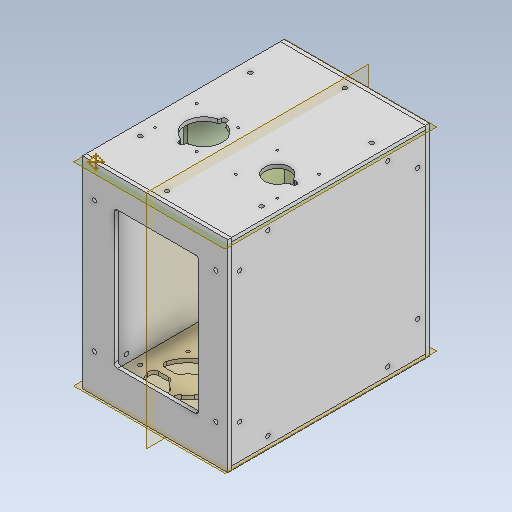
# Autodesk Inventor part: Front face
Saved by Autodesk Inventor 2020 (Build 240168000, 168)
## iProperties
Created: 2020-04-08
Part Number: Front face
Material: Generic
Document SubType Name: Modeling
Designer: angusaitken
Density: 1 g/cm^3
Appearance: Default
Author: angusaitken
Autodesk Inventor part; units mm, degrees
ref_plane "YZ Plane" through (0, 0, 0) normal (1, 0, 0) x (0, 1, 0)
ref_plane "XZ Plane" through (0, 0, 0) normal (0, 1, 0) x (-1, 0, 0)
sketch "Sketch1" plane through (0, 0, 0) normal (0, 0, 1) x (1, 0, 0)
  line L0 (0, 0) -> (170.5, 0)
  line L1 (170.5, 0) -> (170.5, 240.5)
  line L2 (170.5, 240.5) -> (0, 240.5)
  line L3 (0, 240.5) -> (0, 0)
  line L4 (175.25, 245.25) -> (175.25, -4.75)
  line L5 (175.25, -4.75) -> (-4.75, -4.75)
  line L6 (-4.75, -4.75) -> (-4.75, 245.25)
  line L7 (-4.75, 245.25) -> (175.25, 245.25)
  line L8 (137.1, 204.87) -> (137.1, 42.67) projected
  line L9 (137.1, 204.87) -> (137.1, 42.67) projected
  arc A0 (137.1, 204.87) -> (135.1, 206.87) centre (135.1, 204.87) ccw projected
  line L10 (38.5, 206.87) -> (135.1, 206.87) projected
  arc A1 (38.5, 206.87) -> (36.5, 204.87) centre (38.5, 204.87) ccw projected
  line L11 (36.5, 42.67) -> (36.5, 204.87) projected
  arc A2 (36.5, 42.67) -> (38.5, 40.67) centre (38.5, 42.67) ccw projected
  line L12 (135.1, 40.67) -> (38.5, 40.67) projected
  arc A3 (135.1, 40.67) -> (137.1, 42.67) centre (135.1, 42.67) ccw projected
  arc A4 (139.1, 204.87) -> (135.1, 208.87) centre (135.1, 204.87) ccw
  line L13 (135.1, 208.87) -> (38.5, 208.87)
  arc A5 (38.5, 208.87) -> (34.5, 204.87) centre (38.5, 204.87) ccw
  line L14 (34.5, 204.87) -> (34.5, 42.67)
  arc A6 (34.5, 42.67) -> (38.5, 38.67) centre (38.5, 42.67) ccw
  line L15 (38.5, 38.67) -> (135.1, 38.67)
  arc A7 (135.1, 38.67) -> (139.1, 42.67) centre (135.1, 42.67) ccw
  line L16 (139.1, 204.87) -> (139.1, 42.67)
  dimension "d0" = 170.5
  dimension "d1" = 240.5
  dimension "d2" = 4.75
  dimension "d5" = 2
  dimension "d6" = 2
  constraints: 24 end point, 8 point on circle, 5 parallel, 4 centre point, 2 perpendicular, 1 horizontal, 9 other
  measures "d0" distance of L2.end L1.end
  measures "d1" distance of L1.end L0.end
  measures "d2" distance between parallel lines of L1 L4
  measures "d5" distance between parallel lines of L10 L13
  measures "d6" distance between parallel lines of L8 L16
extrude "Extrusion1" add sketch "Sketch1" along normal blind 4.75 contours L3 L2 L1 L0 | L4 L5 L6 L7 | L8 A3 L12 A2 L11 A1 L10 A0 | L16 A7 L15 A6 L14 A5 L13 A4
sketch "Sketch2" plane through (0, 0, 0) normal (0, 0, -1) x (-1, 0, 0)
  line L0 (-137.1, 204.87) -> (-137.1, 42.67) projected
  line L1 (-137.1, 204.87) -> (-137.1, 42.67) projected
  line L2 (-137.1, 204.87) -> (-137.1, 42.67) projected
  arc A0 (-135.1, 206.87) -> (-137.1, 204.87) centre (-135.1, 204.87) ccw projected
  line L3 (-38.5, 206.87) -> (-135.1, 206.87) projected
  arc A1 (-36.5, 204.87) -> (-38.5, 206.87) centre (-38.5, 204.87) ccw projected
  line L4 (-36.5, 42.67) -> (-36.5, 204.87) projected
  arc A2 (-38.5, 40.67) -> (-36.5, 42.67) centre (-38.5, 42.67) ccw projected
  line L5 (-135.1, 40.67) -> (-38.5, 40.67) projected
  arc A3 (-137.1, 42.67) -> (-135.1, 40.67) centre (-135.1, 42.67) ccw projected
  line L6 (-139.1, 204.87) -> (-139.1, 42.67)
  arc A4 (-135.1, 208.87) -> (-139.1, 204.87) centre (-135.1, 204.87) ccw
  line L7 (-135.1, 208.87) -> (-38.5, 208.87)
  arc A5 (-34.5, 204.87) -> (-38.5, 208.87) centre (-38.5, 204.87) ccw
  line L8 (-34.5, 204.87) -> (-34.5, 42.67)
  arc A6 (-38.5, 38.67) -> (-34.5, 42.67) centre (-38.5, 42.67) ccw
  line L9 (-38.5, 38.67) -> (-135.1, 38.67)
  arc A7 (-139.1, 42.67) -> (-135.1, 38.67) centre (-135.1, 42.67) ccw
  point P0 (0, 0)
  point P1 (-139.1, 204.87)
  dimension "d9" = 2
  dimension "d10" = 2
  constraints: 8 end point, 8 point on circle, 4 centre point, 1 parallel, 6 other
  measures "d9" distance between parallel lines of L0 L6
  measures "d10" distance between parallel lines of L3 L7
extrude "Extrusion2" cut sketch "Sketch2" against normal through all contours A0 L3 A1 L4 A2 L5 A3 L0 | A4 L7 A5 L8 A6 L9 A7 L6
sketch "Sketch3" plane through (0, 0, 0) normal (0, 0, -1) x (-1, 0, 0)
  line L0 (-135.1, 208.87) -> (-38.5, 208.87) projected
  arc A0 (-34.5, 204.87) -> (-38.5, 208.87) centre (-38.5, 204.87) ccw projected
  line L1 (-34.5, 204.87) -> (-34.5, 42.67) projected
  arc A1 (-38.5, 38.67) -> (-34.5, 42.67) centre (-38.5, 42.67) ccw projected
  line L2 (-38.5, 38.67) -> (-135.1, 38.67) projected
  arc A2 (-139.1, 42.67) -> (-135.1, 38.67) centre (-135.1, 42.67) ccw projected
  line L3 (-139.1, 42.67) -> (-139.1, 204.87) projected
  arc A3 (-135.1, 208.87) -> (-139.1, 204.87) centre (-135.1, 204.87) ccw projected
  line L4 (4.75, -4.75) -> (-175.25, -4.75) projected
  line L5 (4.75, 245.25) -> (4.75, -4.75) projected
  line L6 (-175.25, 245.25) -> (4.75, 245.25) projected
  line L7 (-175.25, -4.75) -> (-175.25, 245.25) projected
  line L8 (-170.5, 240.5) -> (0, 240.5)
  line L9 (0, 240.5) -> (0, 0)
  line L10 (0, 0) -> (-170.5, 0)
  line L11 (-170.5, 0) -> (-170.5, 240.5)
  point P0 (0, 0)
  dimension "d11" = 4.75
  constraints: 8 end point, 3 other
  measures "d11" distance between parallel lines of L7 L11
ref_plane "Work Plane1" through (152.5168, 19.9337, -238.5381) normal (0, 0, -1) x (0, 1, 0)
extrude "Extrusion3" add sketch "Sketch3" along normal up to surface (238.5381 mm away) separate body contours L4 L7 L6 L5
ref_plane "Work Plane2" through (0, 240.5, 0) normal (0, -1, 0) x (1, 0, 0)
split body "Split1" result two bodies by plane through (0, 240.5, 0) normal (0, -1, 0) bodies 2 first body at (174.75, 158.75, -159.0254)
ref_plane "Work Plane3" through (0, 0, 0) normal (0, 1, 0) x (1, 0, 0)
split body "Split2" result two bodies by plane through (0, 0, 0) normal (0, 1, 0) bodies 3 first body at (174.75, 160.3333, -79.5127) (-0.5, 160.3333, -79.5127)
sketch "Sketch4" plane through (175.25, 240.5, -238.5381) normal (0, 0, -1) x (-1, 0, 0)
  line L0 (40.15, -31.63) -> (136.75, -31.63) projected
  arc A0 (140.75, -35.63) -> (136.75, -31.63) centre (136.75, -35.63) ccw projected
  line L1 (140.75, -35.63) -> (140.75, -197.83) projected
  arc A1 (136.75, -201.83) -> (140.75, -197.83) centre (136.75, -197.83) ccw projected
  line L2 (136.75, -201.83) -> (40.15, -201.83) projected
  arc A2 (36.15, -197.83) -> (40.15, -201.83) centre (40.15, -197.83) ccw projected
  line L3 (36.15, -197.83) -> (36.15, -35.63) projected
  arc A3 (40.15, -31.63) -> (36.15, -35.63) centre (40.15, -35.63) ccw projected
  line L4 (180, -245.25) -> (0, -245.25) projected
  line L5 (180, 4.75) -> (180, -245.25) projected
  line L6 (0, 4.75) -> (180, 4.75) projected
  line L7 (0, -245.25) -> (0, 4.75) projected
  point P0 (175.25, -240.5)
extrude "Extrusion4" add sketch "Sketch4" along normal blind 4.75 separate body contours L0 A0 L1 A1 L2 A2 L3 A3 | L4 L7 L6 L5
sketch "Sketch5" plane through (0, 0, 4.75) normal (0, 0, 1) x (1, 0, 0)
  line L0 (38.5, 208.87) -> (135.1, 208.87) projected
  arc A0 (139.1, 204.87) -> (135.1, 208.87) centre (135.1, 204.87) ccw projected
  line L1 (139.1, 204.87) -> (139.1, 42.67) projected
  arc A1 (135.1, 38.67) -> (139.1, 42.67) centre (135.1, 42.67) ccw projected
  line L2 (135.1, 38.67) -> (38.5, 38.67) projected
  arc A2 (34.5, 42.67) -> (38.5, 38.67) centre (38.5, 42.67) ccw projected
  line L3 (34.5, 42.67) -> (34.5, 204.87) projected
  arc A3 (38.5, 208.87) -> (34.5, 204.87) centre (38.5, 204.87) ccw projected
  line L4 (-4.75, -4.75) -> (175.25, -4.75) projected
  line L5 (175.25, -4.75) -> (175.25, 245.25) projected
  line L6 (175.25, 245.25) -> (-4.75, 245.25) projected
  line L7 (-4.75, 245.25) -> (-4.75, -4.75) projected
  line L8 (10, 10) -> (160.5, 10)
  line L9 (160.5, 10) -> (160.5, 230.5)
  line L10 (160.5, 230.5) -> (10, 230.5)
  line L11 (10, 230.5) -> (10, 10)
  circle A4 centre (10, 204.87) radius 2.6
  circle A5 centre (160.5, 204.87) radius 2.6
  circle A6 centre (10, 42.67) radius 2.6
  circle A7 centre (160.5, 42.67) radius 2.6
  point P0 (0, 0)
  dimension "d18" = 14.75
  dimension "d19" = 5.2
  dimension "d20" = 5.2
  dimension "d21" = 5.2
  dimension "d22" = 5.2
  constraints: 8 end point, 4 centre point, 4 point on line, 3 other
  measures "d18" distance between parallel lines of L7 L11
  measures "d19" diameter of A4
  measures "d20" diameter of A5
  measures "d21" diameter of A6
  measures "d22" diameter of A7
extrude "Extrusion5" cut sketch "Sketch5" against normal through all contours A6 L11 | L11 A6 | A7 L9 | L9 A7 | A4 L11 | L11 A4 | A5 L9 | L9 A5 bodies 1 7
sketch "Sketch6" plane through (-4.75, 240.5, -238.5381) normal (-1, 0, 0) x (0, 0, 1)
  line L0 (0, 0) -> (0, -240.5) projected
  line L1 (238.5381, -240.5) -> (0, -240.5) projected
  line L2 (238.5381, -240.5) -> (238.5381, 0) projected
  line L3 (0, 0) -> (238.5381, 0) projected
  line L4 (0, 0) -> (0, -240.5) projected
  line L5 (228.5381, -10) -> (228.5381, -230.5)
  line L6 (228.5381, -230.5) -> (10, -230.5)
  line L7 (10, -230.5) -> (10, -10)
  line L8 (10, -10) -> (228.5381, -10)
  line L9 (243.2881, -33.03) -> (243.2881, -38.23) projected
  line L10 (243.2881, -195.23) -> (243.2881, -200.43) projected
  circle A0 centre (228.5381, -35.63) radius 2.6
  circle A1 centre (228.5381, -197.83) radius 2.6
  circle A2 centre (10, -197.83) radius 2.6
  circle A3 centre (10, -35.63) radius 2.6
  circle A4 centre (45, -230.5) radius 2.6
  circle A5 centre (193.5381, -230.5) radius 2.6
  circle A6 centre (45, -10) radius 2.6
  circle A7 centre (193.5381, -10) radius 2.6
  point P0 (238.5381, -240.5)
  point P1 (119.269, -120.25)
  dimension "d25" = 10
  dimension "d26" = 5.2
  dimension "d27" = 5.2
  dimension "d28" = 5.2
  dimension "d29" = 5.2
  dimension "d30" = 5.2
  dimension "d31" = 5.2
  dimension "d32" = 35
  dimension "d33" = 35
  dimension "d34" = 5.2
  dimension "d35" = 5.2
  constraints: 8 centre point, 8 end point, 6 point on line, 3 other
  measures "d25" distance between parallel lines of L3 L8
  measures "d26" diameter of A0
  measures "d27" diameter of A1
  measures "d28" diameter of A2
  measures "d29" diameter of A3
  measures "d30" diameter of A4
  measures "d31" diameter of A5
  measures "d32" distance of L6.end A4.centre
  measures "d33" distance of L5.end A5.centre
  measures "d34" diameter of A6
  measures "d35" diameter of A7
extrude "Extrusion6" cut sketch "Sketch6" against normal through all contours A0 L5 | L5 A0 | A7 L8 | L8 A7 | A1 L5 | L5 A1 | A6 L8 | L8 A6 | A5 L6 | L6 A5 | A3 L7 | L7 A3 | A4 L6 | L6 A4 | A2 L7 | L7 A2 bodies 5
move or copy body "Move Body1" bodies to move or copy 7 copy no translate (0, 0, -1.947)
thicken "Thicken1" operation add thickness 1.947 both sides no extend neighbours yes toward (0, 0, -1) bodies 5 faces at (-1.5833, 160.3333, -238.5381)
move faces "Move1" translate (0, 0, -1.947) faces at (113.6667, 243.6667, -238.5381)
move faces "Move2" translate (0, 0, -1.947) faces at (56.8333, -3.1667, -238.5381)
move faces "Move3" translate (0, 0, -1.947) faces at (173.6667, 160.3333, -238.5381)
move faces "Move4" translate (0, 0, -1.947) faces at (172.0833, 40.1727, -229.2615)
move faces "Move5" translate (0, 0, -1.947) faces at (172.0833, 202.3727, -229.2615)
move faces "Move6" translate (0, 0, -1.947) faces at (-1.5833, 202.3727, -229.2615) (-1.5833, 40.1727, -229.2615)
sketch "Sketch7" plane through (-4.75, -4.75, 0) normal (0, -1, 0) x (1, 0, 0)
  circle A0 centre (14.7449, -9.98) radius 4.725
  circle A1 centre (165.2551, -9.98) radius 4.725
  circle A2 centre (165.2551, -230.4902) radius 2.6
  circle A3 centre (14.7449, -230.4902) radius 2.6
  point P0 (4.75, 0)
  constraints: 4 centre point, 8 other
hole "Hole1" at (160.5051, -4.75, -9.98) at (9.9949, -4.75, -9.98) at (9.9949, -4.75, -230.4902) at (160.5051, -4.75, -230.4902) direction (0, 1, 0) diameter 4.2 end through all bodies 6
ref_plane "Work Plane4" through (86.8, 42.67, 0) normal (1, 0, 0) x (0, 0, -1)
sketch "Sketch10" plane through (175.25, 245.25, -245.2351) normal (0, 0, -1) x (-1, 0, 0)
  circle A0 centre (85.2205, -159.8102) radius 42.45
  circle A1 centre (85.2205, -107.3602) radius 2.4
  circle A2 centre (39.7975, -186.0352) radius 2.4
  circle A3 centre (130.6435, -186.0352) radius 2.4
  point P0 (175.25, -245.25)
  constraints: 4 centre point, 8 other
extrude "Extrusion9" cut sketch "Sketch10" against normal through all bodies 7
sketch "Sketch11" plane through (-4.75, 0, 0) normal (-1, 0, 0) x (0, 0, 1)
  arc A0 (-158.1352, 97.3397) -> (-162.885, 92.5899) centre (-158.1352, 92.5899) ccw
  line L0 (-158.1352, 97.3397) -> (-143.835, 97.3397)
  arc A1 (-139.0852, 92.5899) -> (-143.835, 97.3397) centre (-143.835, 92.5899) ccw
  line L1 (-139.0852, 92.5899) -> (-139.0852, 78.2897)
  arc A2 (-143.835, 73.5399) -> (-139.0852, 78.2897) centre (-143.835, 78.2897) ccw
  line L2 (-143.835, 73.5399) -> (-158.1352, 73.5399)
  arc A3 (-162.885, 78.2897) -> (-158.1352, 73.5399) centre (-158.1352, 78.2897) ccw
  line L3 (-162.885, 78.2897) -> (-162.885, 92.5899)
  line L4 (-143.835, 97.8397) -> (-158.1352, 97.8397)
  arc A4 (-158.1352, 97.8397) -> (-163.385, 92.5899) centre (-158.1352, 92.5899) ccw
  line L5 (-163.385, 92.5899) -> (-163.385, 78.2897)
  arc A5 (-163.385, 78.2897) -> (-158.1352, 73.0399) centre (-158.1352, 78.2897) ccw
  line L6 (-158.1352, 73.0399) -> (-143.835, 73.0399)
  arc A6 (-143.835, 73.0399) -> (-138.5852, 78.2897) centre (-143.835, 78.2897) ccw
  line L7 (-138.5852, 78.2897) -> (-138.5852, 92.5899)
  arc A7 (-138.5852, 92.5899) -> (-143.835, 97.8397) centre (-143.835, 92.5899) ccw
  point P0 (0, 0)
  dimension "d79" = 0.5
  constraints: 16 end point, 16 point on circle, 8 centre point, 27 other
  measures "d79" distance between parallel lines of L0 L4
extrude "Extrusion10" cut sketch "Sketch11" against normal blind 10 contours L0 A1 L1 A2 L2 A3 L3 A0 | A7 L7 A6 L6 A5 L5 A4 L4 bodies 5
sketch "Sketch12" plane through (-4.75, 0, 0) normal (-1, 0, 0) x (0, 0, 1)
  line L0 (-120.9351, 195.1795) -> (-120.9351, 219.9795)
  line L1 (-120.9351, 219.9795) -> (-68.5351, 219.9795)
  line L2 (-68.5351, 219.9795) -> (-68.5351, 195.1795)
  line L3 (-68.5351, 195.1795) -> (-120.9351, 195.1795)
  point P0 (0, 0)
  constraints: 8 end point, 2 horizontal, 2 vertical, 4 other
extrude "Extrusion11" cut sketch "Sketch12" against normal blind 10 bodies 5
sketch "Sketch13" plane through (-4.75, 245.25, 0) normal (0, 1, 0) x (1, 0, 0)
  circle A0 centre (39.495, 94.7351) radius 12.65
  circle A1 centre (140.5, 94.7351) radius 12.65
  point P0 (4.75, 0)
  constraints: 2 centre point, 4 other
hole "Hole2" at (34.745, 245.25, -94.7351) at (135.75, 245.25, -94.7351) direction (0, -1, 0) diameter 31 end through all bodies 4
sketch "Sketch14" plane through (-4.75, 245.25, 0) normal (0, 1, 0) x (1, 0, 0)
  circle A0 centre (65.245, 68.9851) radius 1.6
  circle A1 centre (13.745, 68.9851) radius 1.6
  circle A2 centre (65.245, 120.4851) radius 1.6
  circle A3 centre (13.745, 120.4851) radius 1.6
  circle A4 centre (166.25, 120.4851) radius 1.6
  circle A5 centre (114.75, 120.4851) radius 1.6
  circle A6 centre (114.75, 68.9851) radius 1.6
  circle A7 centre (166.25, 68.9851) radius 1.6
  point P0 (4.75, 0)
  constraints: 8 centre point, 16 other
hole "Hole3" at (8.995, 245.25, -120.4851) at (60.495, 245.25, -120.4851) at (60.495, 245.25, -68.9851) at (8.995, 245.25, -68.9851) at (110, 245.25, -68.9851) at (161.5, 245.25, -68.9851) at (161.5, 245.25, -120.4851) at (110, 245.25, -120.4851) direction (0, -1, 0) diameter 2.8 end through all bodies 4
sketch "Sketch15" plane through (-4.75, 245.25, 0) normal (0, 1, 0) x (1, 0, 0)
  circle A0 centre (160.7871, 95.5911) radius 2.1
  line L0 (160.7871, 95.5911) -> (150.7871, 95.5911) construction
  line L1 (160.7871, 98.7156) -> (150.7871, 98.7156)
  line L2 (150.7871, 92.4666) -> (160.7871, 92.4666)
  arc A1 (160.7871, 92.4666) -> (160.7871, 98.7156) centre (160.7871, 95.5911) ccw
  arc A2 (150.7871, 98.7156) -> (150.7871, 92.4666) centre (150.7871, 95.5911) ccw
  point P0 (4.75, 0)
  point P1 (155.7871, 95.5911)
  dimension "d98" = 10
  constraints: 8 end point, 4 point on circle, 4 tangent, 3 centre point, 1 horizontal, 1 midpoint, 1 parallel, 2 other
  measures "d98" distance of L0.start L0.end
extrude "Extrusion12" cut sketch "Sketch15" against normal blind 10 contours A0 | A1 L2 A2 L1 bodies 4
fillet "Fillet1" radius 4 2 edges at (150.7302, 242.875, -98.7156) (151.0831, 242.875, -92.4666)
sketch "Sketch16" plane through (-4.75, -4.75, 0) normal (0, -1, 0) x (1, 0, 0)
  circle A0 centre (30.018, -96.0748) radius 2.5
  circle A1 centre (30.018, -24.5748) radius 2.5
  circle A2 centre (101.518, -24.5748) radius 2.5
  circle A3 centre (101.518, -96.0748) radius 2.5
  point P0 (4.75, 0)
  constraints: 4 centre point, 8 other
hole "Hole4" at (25.268, -4.75, -96.0748) at (25.268, -4.75, -24.5748) at (96.768, -4.75, -24.5748) at (96.768, -4.75, -96.0748) direction (0, 1, 0) diameter 4 depth 8 bodies 6
sketch "Sketch17" plane through (-4.75, -4.75, 0) normal (0, -1, 0) x (1, 0, 0)
  circle A0 centre (65.768, -60.3248) radius 16.5
  circle A1 centre (65.768, -60.3248) radius 40
  line L0 (69.4761, -18.6373) -> (62.0599, -18.6373)
  line L1 (62.0599, -18.6373) -> (62.0599, -102.0123)
  line L2 (62.0599, -102.0123) -> (69.4761, -102.0123)
  line L3 (69.4761, -102.0123) -> (69.4761, -18.6373)
  line L4 (69.4761, -18.6373) -> (62.0599, -102.0123) construction
  line L5 (62.0599, -18.6373) -> (69.4761, -102.0123) construction
  line L6 (22.784, -64.3248) -> (108.7521, -64.3248)
  line L7 (108.7521, -64.3248) -> (108.7521, -56.3248)
  line L8 (108.7521, -56.3248) -> (22.784, -56.3248)
  line L9 (22.784, -56.3248) -> (22.784, -64.3248)
  line L10 (22.784, -64.3248) -> (108.7521, -56.3248) construction
  line L11 (108.7521, -64.3248) -> (22.784, -56.3248) construction
  point P0 (4.75, 0)
  point P1 (49.7602, -64.3248)
  point P2 (25.9685, -64.3248)
  point P3 (62.0599, -100.1526)
  point P4 (62.0599, -76.4027)
  point P5 (105.5675, -64.3248)
  point P6 (81.7758, -64.3248)
  point P7 (69.4761, -76.4027)
  point P8 (69.4761, -100.1526)
  point P9 (81.7758, -56.3248)
  point P10 (105.5675, -56.3248)
  point P11 (69.4761, -20.4971)
  point P12 (69.4761, -44.2469)
  point P13 (25.9685, -56.3248)
  point P14 (49.7602, -56.3248)
  point P15 (62.0599, -44.2469)
  point P16 (62.0599, -20.4971)
  dimension "d109" = 80
  dimension "d110" = 8
  constraints: 24 end point, 4 midpoint, 4 parallel, 2 centre point, 2 horizontal, 2 perpendicular, 1 coincident, 2 other
  measures "d109" diameter of A1
  measures "d110" distance of L7.end L6.end
extrude "Extrusion13" cut sketch "Sketch17" against normal through all contours A0 L3 A1 L8 | L6 A1 L3 A0 | A0 L8 A1 L1 | L1 A1 L6 A0 bodies 6
fillet "Fillet2" radius 6 16 edges at (64.7261, -2.375, -44.2469) (64.7261, -2.375, -20.4971) (77.0258, -2.375, -56.3248) (100.8175, -2.375, -56.3248) (100.8175, -2.375, -64.3248) (77.0258, -2.375, -64.3248) (64.7261, -2.375, -76.4027) (57.3099, -2.375, -76.4027) (45.0102, -2.375, -64.3248) (45.0102, -2.375, -56.3248) (57.3099, -2.375, -44.2469) (57.3099, -2.375, -20.4971) (21.2185, -2.375, -56.3248) (21.2185, -2.375, -64.3248) (57.3099, -2.375, -100.1526) (64.7261, -2.375, -100.1526)
sketch "Sketch18" plane through (-4.75, 0, 0) normal (-1, 0, 0) x (0, 0, 1)
  circle A0 centre (-216.8953, 37.4898) radius 1.7
  circle A1 centre (-180.8953, 37.4898) radius 1.7
  line L0 (-216.8953, 37.4898) -> (-180.8953, 37.4898)
  line L1 (-211.5453, 21.7898) -> (-186.2453, 21.7898)
  line L2 (-185.2453, 22.7898) -> (-185.2453, 52.1898)
  line L3 (-186.2453, 53.1898) -> (-211.5453, 53.1898)
  line L4 (-212.5453, 52.1898) -> (-212.5453, 22.7898)
  line L5 (-212.5453, 21.7898) -> (-185.2453, 53.1898) construction
  line L6 (-185.2453, 21.7898) -> (-212.5453, 53.1898) construction
  arc A2 (-211.5453, 53.1898) -> (-212.5453, 52.1898) centre (-211.5453, 52.1898) ccw
  arc A3 (-212.5453, 22.7898) -> (-211.5453, 21.7898) centre (-211.5453, 22.7898) ccw
  arc A4 (-186.2453, 21.7898) -> (-185.2453, 22.7898) centre (-186.2453, 22.7898) ccw
  arc A5 (-185.2453, 52.1898) -> (-186.2453, 53.1898) centre (-186.2453, 52.1898) ccw
  point P0 (0, 0)
  point P1 (-198.8953, 37.4898)
  dimension "d114" = 27.3
  dimension "d115" = 31.4
  dimension "d116" = 1
  constraints: 14 end point, 8 point on circle, 8 point on line, 8 tangent, 6 centre point, 3 equal radius, 3 midpoint, 2 horizontal, 2 parallel, 1 perpendicular, 4 other
  measures "d114" distance of L6.end L5.end
  measures "d115" distance of L5.end L6.start
  measures "d116" radius of A2
extrude "Extrusion14" cut sketch "Sketch18" against normal blind 10 bodies 5
sketch "Sketch19" plane through (175.25, 245.25, -245.2351) normal (0, 0, -1) x (-1, 0, 0)
  spline S0 degree 3 poles (133.1037, -75.5722) (133.1023, -75.5752) (133.1009, -75.5782) (133.0994, -75.5813) (133.0898, -75.6017) (133.0639, -75.6566) (132.9397, -75.9317) (132.7918, -76.2658) (132.4259, -77.3189) (132.201, -78.1035) (131.9411, -80.0106) (131.9109, -81.1284) (132.2641, -83.7391) (132.7511, -85.2355) (133.504, -86.5725) knots 0.020688 0.020688 0.020688 0.020688 0.041317 0.041317 0.041317 0.18118 0.18118 0.471068 0.471068 0.816157 0.816157 1.156169 1.156169 1.578148 1.578148 1.578148 1.578148
  circle A0 centre (143.9602, -80.6846) radius 3.5
  point P0 (175.25, -245.25)
  constraints: 1 centre point, 6 other
hole "Hole5" at (31.2898, 164.5654, -245.2351) direction (0, 0, 1) diameter 12.7 end through all bodies 7
sketch "Sketch20" plane through (-4.75, 245.25, 0) normal (0, 1, 0) x (1, 0, 0)
  circle A0 centre (49.495, 96.2351) radius 12.65
  circle A1 centre (39.495, 94.7351) radius 15.5 projected
  point P0 (4.75, 0)
  constraints: 1 centre point, 2 other
hole "Hole6" at (44.745, 245.25, -96.2351) direction (0, -1, 0) diameter 32 end through all bodies 4
delete faces "Delete Face1" heal yes whole lump no faces at (40.0049, 243.6667, -80.1548)
sketch "Sketch21" plane through (-4.75, -4.75, 0) normal (0, -1, 0) x (1, 0, 0)
  line L0 (0, 0) -> (0, -240.4851) projected
  line L1 (180, -240.4851) -> (0, -240.4851) projected
  line L2 (180, 0) -> (180, -240.4851) projected
  line L3 (0, 0) -> (180, 0) projected
  circle A0 centre (165.2551, -9.98) radius 2.1 projected
  circle A1 centre (165.2551, -230.4902) radius 2.1 projected
  circle A2 centre (14.7449, -230.4902) radius 2.1 projected
  circle A3 centre (14.7449, -9.98) radius 2.1 projected
  line L4 (25.0343, -149.3857) -> (155.0343, -149.3857)
  line L5 (155.0343, -149.3857) -> (155.0343, -219.3857)
  line L6 (155.0343, -219.3857) -> (25.0343, -219.3857)
  line L7 (25.0343, -219.3857) -> (25.0343, -149.3857)
  line L8 (28.0343, -152.3857) -> (152.0343, -152.3857) construction
  line L9 (152.0343, -152.3857) -> (152.0343, -216.3857) construction
  line L10 (152.0343, -216.3857) -> (28.0343, -216.3857) construction
  line L11 (28.0343, -216.3857) -> (28.0343, -152.3857) construction
  line L12 (28.0343, -152.3857) -> (92.0343, -216.3857) construction
  line L13 (26.9029, -153.5171) -> (90.9029, -217.5171)
  line L14 (93.1656, -215.2543) -> (29.1656, -151.2543)
  arc A4 (29.1656, -151.2543) -> (26.9029, -153.5171) centre (28.0343, -152.3857) ccw
  arc A5 (90.9029, -217.5171) -> (93.1656, -215.2543) centre (92.0343, -216.3857) ccw
  line L15 (28.0343, -152.3857) -> (118.5439, -152.3857) construction
  line L16 (36.9029, -153.5171) -> (100.9029, -217.5171)
  line L17 (103.1656, -215.2543) -> (39.1656, -151.2543)
  arc A6 (100.9029, -217.5171) -> (103.1656, -215.2543) centre (102.0343, -216.3857) ccw
  arc A7 (39.1656, -151.2543) -> (36.9029, -153.5171) centre (38.0343, -152.3857) ccw
  line L18 (46.9029, -153.5171) -> (110.9029, -217.5171)
  line L19 (113.1656, -215.2543) -> (49.1656, -151.2543)
  arc A8 (110.9029, -217.5171) -> (113.1656, -215.2543) centre (112.0343, -216.3857) ccw
  arc A9 (49.1656, -151.2543) -> (46.9029, -153.5171) centre (48.0343, -152.3857) ccw
  line L20 (56.9029, -153.5171) -> (120.9029, -217.5171)
  line L21 (123.1656, -215.2543) -> (59.1656, -151.2543)
  arc A10 (120.9029, -217.5171) -> (123.1656, -215.2543) centre (122.0343, -216.3857) ccw
  arc A11 (59.1656, -151.2543) -> (56.9029, -153.5171) centre (58.0343, -152.3857) ccw
  line L22 (66.9029, -153.5171) -> (130.9029, -217.5171)
  line L23 (133.1656, -215.2543) -> (69.1656, -151.2543)
  arc A12 (130.9029, -217.5171) -> (133.1656, -215.2543) centre (132.0343, -216.3857) ccw
  arc A13 (69.1656, -151.2543) -> (66.9029, -153.5171) centre (68.0343, -152.3857) ccw
  line L24 (76.9029, -153.5171) -> (140.9029, -217.5171)
  line L25 (143.1656, -215.2543) -> (79.1656, -151.2543)
  arc A14 (140.9029, -217.5171) -> (143.1656, -215.2543) centre (142.0343, -216.3857) ccw
  arc A15 (79.1656, -151.2543) -> (76.9029, -153.5171) centre (78.0343, -152.3857) ccw
  line L26 (86.9029, -153.5171) -> (150.9029, -217.5171)
  line L27 (153.1656, -215.2543) -> (89.1656, -151.2543)
  arc A16 (150.9029, -217.5171) -> (153.1656, -215.2543) centre (152.0343, -216.3857) ccw
  arc A17 (89.1656, -151.2543) -> (86.9029, -153.5171) centre (88.0343, -152.3857) ccw
  line L28 (92.0343, -216.3857) -> (82.0343, -216.3857)
  line L29 (82.0343, -216.3857) -> (72.0343, -216.3857)
  line L30 (72.0343, -216.3857) -> (62.0343, -216.3857)
  line L31 (62.0343, -216.3857) -> (52.0343, -216.3857)
  line L32 (52.0343, -216.3857) -> (42.0343, -216.3857)
  line L33 (42.0343, -216.3857) -> (32.0343, -216.3857)
  line L34 (82.0343, -216.3857) -> (28.0343, -162.3857) construction
  line L35 (83.1656, -215.2543) -> (29.1656, -161.2543)
  line L36 (26.9029, -163.5171) -> (80.9029, -217.5171)
  arc A18 (80.9029, -217.5171) -> (83.1656, -215.2543) centre (82.0343, -216.3857) ccw
  arc A19 (29.1656, -161.2543) -> (26.9029, -163.5171) centre (28.0343, -162.3857) ccw
  line L37 (82.0343, -216.3857) -> (158.4018, -216.3857) construction
  line L38 (72.0343, -216.3857) -> (28.0343, -172.3857) construction
  line L39 (73.1656, -215.2543) -> (29.1656, -171.2543)
  line L40 (26.9029, -173.5171) -> (70.9029, -217.5171)
  arc A20 (70.9029, -217.5171) -> (73.1656, -215.2543) centre (72.0343, -216.3857) ccw
  arc A21 (29.1656, -171.2543) -> (26.9029, -173.5171) centre (28.0343, -172.3857) ccw
  line L41 (62.0343, -216.3857) -> (28.0343, -182.3857) construction
  line L42 (63.1656, -215.2543) -> (29.1656, -181.2543)
  line L43 (26.9029, -183.5171) -> (60.9029, -217.5171)
  arc A22 (60.9029, -217.5171) -> (63.1656, -215.2543) centre (62.0343, -216.3857) ccw
  arc A23 (29.1656, -181.2543) -> (26.9029, -183.5171) centre (28.0343, -182.3857) ccw
  line L44 (62.0343, -216.3857) -> (110.1175, -216.3857) construction
  line L45 (52.0343, -216.3857) -> (28.0343, -192.3857) construction
  line L46 (53.1656, -215.2543) -> (29.1656, -191.2543)
  line L47 (26.9029, -193.5171) -> (50.9029, -217.5171)
  arc A24 (50.9029, -217.5171) -> (53.1656, -215.2543) centre (52.0343, -216.3857) ccw
  arc A25 (29.1656, -191.2543) -> (26.9029, -193.5171) centre (28.0343, -192.3857) ccw
  line L48 (42.0343, -216.3857) -> (28.0343, -202.3857) construction
  line L49 (43.1656, -215.2543) -> (29.1656, -201.2543)
  line L50 (26.9029, -203.5171) -> (40.9029, -217.5171)
  arc A26 (40.9029, -217.5171) -> (43.1656, -215.2543) centre (42.0343, -216.3857) ccw
  arc A27 (29.1656, -201.2543) -> (26.9029, -203.5171) centre (28.0343, -202.3857) ccw
  line L51 (32.0343, -216.3857) -> (28.0343, -212.3857) construction
  line L52 (33.1656, -215.2543) -> (29.1656, -211.2543)
  line L53 (26.9029, -213.5171) -> (30.9029, -217.5171)
  arc A28 (30.9029, -217.5171) -> (33.1656, -215.2543) centre (32.0343, -216.3857) ccw
  arc A29 (29.1656, -211.2543) -> (26.9029, -213.5171) centre (28.0343, -212.3857) ccw
  line L54 (90.0343, -149.3857) -> (90.0343, -219.3857) construction
  line L55 (90.0343, -219.3857) -> (90.0343, -149.3857) construction
  line L56 (146.9029, -153.5171) -> (150.9029, -157.5171)
  line L57 (153.1656, -155.2543) -> (149.1656, -151.2543)
  arc A30 (150.9029, -157.5171) -> (153.1656, -155.2543) centre (152.0343, -156.3857) ccw
  arc A31 (150.9029, -167.5171) -> (153.1656, -165.2543) centre (152.0343, -166.3857) ccw
  arc A32 (150.9029, -177.5171) -> (153.1656, -175.2543) centre (152.0343, -176.3857) ccw
  arc A33 (150.9029, -187.5171) -> (153.1656, -185.2543) centre (152.0343, -186.3857) ccw
  arc A34 (150.9029, -197.5171) -> (153.1656, -195.2543) centre (152.0343, -196.3857) ccw
  arc A35 (150.9029, -207.5171) -> (153.1656, -205.2543) centre (152.0343, -206.3857) ccw
  line L58 (96.9029, -153.5171) -> (150.9029, -207.5171)
  line L59 (153.1656, -205.2543) -> (99.1656, -151.2543)
  line L60 (106.9029, -153.5171) -> (150.9029, -197.5171)
  line L61 (153.1656, -195.2543) -> (109.1656, -151.2543)
  line L62 (116.9029, -153.5171) -> (150.9029, -187.5171)
  line L63 (153.1656, -185.2543) -> (119.1656, -151.2543)
  line L64 (126.9029, -153.5171) -> (150.9029, -177.5171)
  line L65 (153.1656, -175.2543) -> (129.1656, -151.2543)
  line L66 (136.9029, -153.5171) -> (150.9029, -167.5171)
  line L67 (153.1656, -165.2543) -> (139.1656, -151.2543)
  arc A36 (149.1656, -151.2543) -> (146.9029, -153.5171) centre (148.0343, -152.3857) ccw
  arc A37 (139.1656, -151.2543) -> (136.9029, -153.5171) centre (138.0343, -152.3857) ccw
  arc A38 (129.1656, -151.2543) -> (126.9029, -153.5171) centre (128.0343, -152.3857) ccw
  arc A39 (119.1656, -151.2543) -> (116.9029, -153.5171) centre (118.0343, -152.3857) ccw
  arc A40 (109.1656, -151.2543) -> (106.9029, -153.5171) centre (108.0343, -152.3857) ccw
  arc A41 (99.1656, -151.2543) -> (96.9029, -153.5171) centre (98.0343, -152.3857) ccw
  point P0 (4.75, 0)
  point P1 (60.0343, -184.3857)
  point P2 (55.0343, -189.3857)
  point P3 (50.0343, -194.3857)
  point P4 (45.0343, -199.3857)
  point P5 (40.0343, -204.3857)
  point P6 (35.0343, -209.3857)
  point P7 (30.0343, -214.3857)
  point P8 (90.0343, -184.3857)
  point P9 (90.0343, -184.3857)
  dimension "d133" = 130
  dimension "d134" = 70
  dimension "d135" = 3
  dimension "d136" = 45
  dimension "d137" = 3.2
  dimension "d140" = 10
  dimension "d145" = 10
  dimension "d146" = 10
  dimension "d147" = 10
  dimension "d148" = 10
  dimension "d149" = 10
  dimension "d150" = 10
  dimension "d151" = 135
  dimension "d152" = 3.2
  dimension "d153" = 3.2
  dimension "d154" = 135
  dimension "d155" = 3.2
  dimension "d158" = 360
  constraints: 140 end point, 76 point on circle, 38 centre point, 36 horizontal alignment, 28 tangent, 26 parallel, 12 equal radius, 10 midpoint, 6 point on line, 5 horizontal, 3 equal length, 2 coincident, 2 perpendicular, 140 other
  measures "d133" distance of L5.end L6.end
  measures "d134" distance of L4.end L5.end
  measures "d135" distance between parallel lines of L7 L11
  measures "d136" angle of L12 L15
  measures "d137" diameter of A5
  measures "d140" distance of L13.start L16.start
  measures "d145" distance of L12.end L28.end
  measures "d146" distance of L28.end L29.end
  measures "d147" distance of L29.end L30.end
  measures "d148" distance of L30.end L31.end
  measures "d149" distance of L31.end L32.end
  measures "d150" distance of L32.end L33.end
  measures "d151" angle of L37 L34
  measures "d152" diameter of A19
  measures "d153" diameter of A21
  measures "d154" angle of L44 L41
  measures "d155" diameter of A23
extrude "Extrusion15" cut sketch "Sketch21" against normal through all contours A4 L14 A5 L13 | A7 L17 A6 L16 | A9 L19 A8 L18 | A11 L21 A10 L20 | A13 L23 A12 L22 | A15 L25 A14 L24 | A17 L27 A16 L26 | A18 L36 L29 L28 | L28 L29 L36 A19 L35 A18 | A20 L40 L30 L29 | L29 L30 L40 A21 L39 A20 | A22 L43 L31 L30 | L30 L31 L43 A23 L42 A22 | A24 L47 L32 L31 | L31 L32 L47 A25 L46 A24 | A26 L50 L33 L32 | L32 L33 L50 A27 L49 A26 | A28 L53 A29 L52 | A36 L57 A30 L56 | L66 A37 L67 A31 | L64 A38 L65 A32 | L62 A39 L63 A33 | L60 A40 L61 A34 | L58 A41 L59 A35 bodies 6
move faces "Move8" translate (0, 0, -1.5) faces at (109.7754, 243.6667, -67.6032) (161.9433, 243.6667, -67.6571) (161.9433, 243.6667, -119.1571) (109.7754, 243.6667, -119.1032) (60.6077, 243.6667, -119.0896) (60.6077, 243.6667, -67.5896) (7.6233, 243.6667, -68.7051) (7.6233, 243.6667, -120.2051)
move faces "Move9" translate (0.889, 0, 0) faces at (60.6077, 243.6667, -69.0896) (7.6233, 243.6667, -70.2051) (7.6233, 243.6667, -121.7051) (60.6077, 243.6667, -120.5896)
sketch "Sketch22" plane through (-4.75, 245.25, 0) normal (0, 1, 0) x (1, 0, 0)
  circle A0 centre (49.495, 121.2351) radius 2
  circle A1 centre (47.0211, 71.2351) radius 2
  point P0 (4.75, 0)
  constraints: 2 centre point, 4 other
extrude "Extrusion16" cut sketch "Sketch22" against normal through all bodies 4
sketch "Sketch23" plane through (-4.75, 245.25, 0) normal (0, 1, 0) x (1, 0, 0)
  circle A0 centre (14.7449, 9.98) radius 2.1463
  circle A1 centre (165.2551, 9.98) radius 2.1463
  circle A2 centre (165.2551, 230.4902) radius 2.1463
  circle A3 centre (14.7449, 230.4902) radius 2.1463
  line L0 (0, 240.4851) -> (180, 240.4851) projected
  line L1 (180, 0) -> (0, 0) projected
  line L2 (167.4013, 10) -> (12.5987, 10)
  line L3 (12.5986, 230.4851) -> (167.4014, 230.4851)
  line L4 (0, 0) -> (0, 240.4851) projected
  line L5 (180, 0) -> (180, 240.4851) projected
  line L6 (165.25, 230.4851) -> (165.25, 10)
  line L7 (14.75, 10) -> (14.75, 230.4851)
  line L8 (167.4013, 52) -> (12.5987, 52)
  line L9 (12.5986, 188.4851) -> (167.4014, 188.4851)
  point P0 (4.75, 0)
  point P1 (14.75, 188.4851)
  point P2 (165.25, 188.4851)
  point P3 (90, 230.4851)
  point P4 (90, 10)
  point P5 (14.75, 52)
  point P6 (165.25, 52)
  dimension "d170" = 10
  dimension "d171" = 10
  dimension "d172" = 14.75
  dimension "d173" = 42
  dimension "d174" = 42
  constraints: 12 end point, 12 point on line, 4 parallel, 2 midpoint, 18 other
  measures "d170" distance between parallel lines of L1 L2
  measures "d171" distance between parallel lines of L0 L3
  measures "d172" distance of the line from the sketch origin of L7
  measures "d173" distance between parallel lines of L2 L8
  measures "d174" distance between parallel lines of L3 L9
hole "Hole7" at (10, 245.25, -188.4851) at (160.5, 245.25, -188.4851) at (85.25, 245.25, -230.4851) at (85.25, 245.25, -10) at (10, 245.25, -52) at (160.5, 245.25, -52) direction (0, -1, 0) diameter 5.2 depth 250 bodies 4 6
move faces "Move10" translate (0, 0, -1.5) faces at (150.1851, 243.6667, -100.5407) (133.8946, 243.6667, -79.3465) (155.2055, 243.6667, -98.7156) (158.4574, 242.0833, -93.615) (153.5548, 243.6667, -92.4117) (154.8224, 243.6667, -92.4666)
sketch "Sketch24" plane through (-4.75, 245.25, 0) normal (0, 1, 0) x (1, 0, 0)
  arc A0 (52.7418, 121.0914) -> (55.0043, 118.0502) centre (55.7389, 120.9588) ccw
  arc A1 (52.7418, 121.0914) -> (46.2482, 121.0914) centre (49.495, 121.2351) ccw
  arc A2 (43.9857, 118.0502) -> (41.8698, 75.0666) centre (49.495, 96.2351) ccw
  arc A3 (43.9857, 118.0502) -> (46.2482, 121.0914) centre (43.2511, 120.9588) ccw
  arc A4 (43.8137, 71.7598) -> (41.8698, 75.0666) centre (40.8531, 72.2441) ccw
  circle A5 centre (47.0211, 71.2351) radius 3.25
  arc A6 (52.8234, 73.9826) -> (55.0043, 118.0502) centre (49.495, 96.2351) ccw
  arc A7 (52.8234, 73.9826) -> (50.2691, 71.121) centre (53.2672, 71.0156) ccw
  point P0 (4.75, 0)
  constraints: 14 point on circle, 8 centre point, 24 other
extrude "Extrusion17" cut sketch "Sketch24" against normal blind 10 bodies 4
offset faces "Size1" outward -0.3 bodies 4 faces at (24.5123, 242.0833, -86.392) (41.1514, 242.0833, -119.5532) (47.7752, 242.0833, -122.41) (49.2281, 242.0833, -118.5299) (61.3455, 242.0833, -111.423) (39.0711, 242.0833, -72.6809) (43.8971, 242.0833, -68.4211) (46.9908, 242.0833, -73.5983)
delete faces "Delete Face2" heal yes whole lump no faces at (31.8008, 170.8948, -242.0684)
sketch "Sketch25" plane through (-4.75, 0, 0) normal (-1, 0, 0) x (0, 0, 1)
  circle A0 centre (-198.1953, 81.7548) radius 3.5
  point P0 (0, 0)
  constraints: 1 centre point, 2 other
hole "Hole8" at (-4.75, 81.7548, -198.1953) direction (1, 0, 0) diameter 12.7 depth 8 bodies 5
equation "\"d20\" = d19"
equation "\"d21\" = d19"
equation "\"d22\" = d19"
equation "\"d33\" = d32"
body "Solid1"
body "Solid7"
body "Solid4"
body "Solid5"
body "Solid6"
